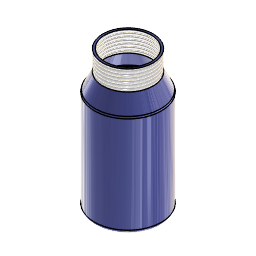
bottle_bottom (Autodesk Fusion 360 archive; units mm, degrees)
design "bottle_bottom" references "hhhhhhh"
part number: 2025-09-29-05-59-28-951
Autodesk Fusion 360 part; units mm, degrees
sketch "Sketch1" plane through (0, 0, 0) normal (0, 0, 1) x (1, 0, 0)
  circle A0 centre (0, 0) radius 16.5
  dimension "d1" = 33
  constraint coincident A0.centre origin
  measures "d1" diameter of A0
extrude "Extrude1" add sketch "Sketch1" along normal blind 50
ref_plane "WorkPlane1" through (0, 0, 55) normal (0, 0, 1) x (1, 0, 0)
sketch "Sketch2" plane through (0, 0, 55) normal (0, 0, 1) x (1, 0, 0)
  circle A0 centre (0, 0) radius 12.5
  dimension "d5" = 25
  constraint coincident A0.centre origin
  measures "d5" diameter of A0
ref_plane "WorkPlane2" through (0, 0, 58) normal (0, 0, 1) x (1, 0, 0)
sketch "Sketch3" plane through (0, 0, 58) normal (0, 0, 1) x (1, 0, 0)
  circle A0 centre (0, 0) radius 12.5
  dimension "d9" = 25
  constraint coincident A0.centre origin
  measures "d9" diameter of A0
loft "Loft2" add profiles "Sketch3" section 1 face at (-4.5443, 3.0983, 50) section 2
extrude "Extrude3" add 1 faces at (-3.3879, -0.621, 58) along direction (0, 0, 1) blind 10
thread "Thread1" "ISO Metric profile 25.0 M25x1.5 M25x1.5 6g" major diameter 24.85 minor diameter 23.132 pitch 1.5 angle 60 resizes the face on face at (12.4845, -0.6231, 64.6667)
fillet "Fillet1" radius 2 2 edges at (-15.3834, -5.9667, 50) (-15.3834, -5.9667, 0)
shell "Shell1" thickness 1 removed faces 1 at (-1.595, 5.7536, 68)

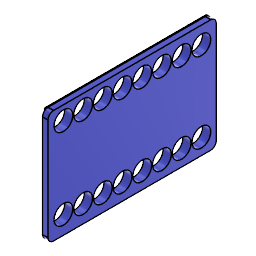
design "hhhhhhh"
part number: 2025-09-26-13-29-13-147
Autodesk Fusion 360 part; units mm, degrees
sketch "Sketch1" plane through (0, 0, 0) normal (1, 0, 0) x (0, 1, 0)
  line L0 (-10, 0) -> (-295, 0)
  line L1 (-305, 10) -> (-305, 195)
  line L2 (-295, 205) -> (-10, 205)
  line L3 (0, 195) -> (0, 10)
  circle A0 centre (-27, 174) radius 17
  circle A1 centre (-62.7143, 175) radius 17
  circle A2 centre (-98.4283, 176) radius 17
  circle A3 centre (-134.1423, 177) radius 17
  circle A4 centre (-169.8563, 178) radius 17
  circle A5 centre (-205.5703, 179) radius 17
  circle A6 centre (-241.2843, 179.5) radius 17
  circle A7 centre (-276.9983, 180) radius 17
  circle A8 centre (-27, 29) radius 17
  circle A9 centre (-62.7127, 29.3029) radius 17
  circle A10 centre (-98.4267, 29.6) radius 17
  circle A11 centre (-134.1407, 29.9) radius 17
  circle A12 centre (-169.8547, 30.1) radius 17
  circle A13 centre (-205.5687, 31) radius 17
  circle A14 centre (-241.2827, 32) radius 17
  arc A15 (-305, 10) -> (-295, 0) centre (-295, 10) ccw
  arc A16 (-295, 205) -> (-305, 195) centre (-295, 195) ccw
  arc A17 (0, 195) -> (-10, 205) centre (-10, 195) ccw
  arc A18 (-10, 0) -> (0, 10) centre (-10, 10) ccw
  circle A19 centre (-276.9967, 33) radius 17
  dimension "d1" = 305
  dimension "d2" = 205
  dimension "d3" = 34
  dimension "d4" = 27
  dimension "d5" = 31
  dimension "d6" = 34
  dimension "d7" = 34
  dimension "d8" = 34
  dimension "d9" = 34
  dimension "d10" = 34
  dimension "d11" = 35.7143
  dimension "d12" = 35.714
  dimension "d13" = 35.714
  dimension "d14" = 35.714
  dimension "d15" = 35.714
  dimension "d16" = 34
  dimension "d17" = 34
  dimension "d18" = 35.714
  dimension "d19" = 35.714
  dimension "d20" = 28.0017
  dimension "d21" = 34
  dimension "d22" = 34
  dimension "d23" = 34
  dimension "d24" = 34
  dimension "d25" = 34
  dimension "d26" = 34
  dimension "d27" = 34
  dimension "d28" = 27
  dimension "d29" = 35.714
  dimension "d30" = 35.714
  dimension "d31" = 10
  dimension "d32" = 10
  dimension "d33" = 10
  dimension "d34" = 10
  dimension "d35" = 35.714
  dimension "d36" = 35.714
  dimension "d37" = 35.714
  dimension "d38" = 35.714
  dimension "d39" = 34
  dimension "d40" = 35.714
  dimension "d41" = 28.0033
  dimension "d42" = 29
  dimension "d44" = 29.6
  dimension "d45" = 29.3029
  dimension "d46" = 29.9
  dimension "d47" = 30.1
  dimension "d48" = 31
  dimension "d49" = 32
  dimension "d50" = 33
  dimension "d51" = 25
  dimension "d52" = 25.5
  dimension "d53" = 26
  dimension "d54" = 27
  dimension "d55" = 28
  dimension "d56" = 29
  dimension "d57" = 30
  dimension "d58" = 31
  constraint horizontal L0
  constraint vertical L1
  constraint horizontal L2
  constraint vertical L3
  constraint tangent L0 A15
  constraint tangent L1 A15
  constraint tangent L1 A16
  constraint tangent L2 A16
  constraint tangent L3 A17
  constraint tangent L2 A17
  constraint tangent L0 A18
  constraint tangent L3 A18
  measures "d1" distance of L1 L3
  measures "d2" distance of L0 L2
  measures "d3" diameter of A0
  measures "d4" distance of L3 A0.centre
  measures "d5" distance of L2 A0.centre
  measures "d6" diameter of A1
  measures "d7" diameter of A2
  measures "d8" diameter of A3
  measures "d9" diameter of A4
  measures "d10" diameter of A5
  measures "d11" horizontal distance of A0.centre A1.centre
  measures "d12" horizontal distance of A1.centre A2.centre
  measures "d13" horizontal distance of A2.centre A3.centre
  measures "d14" horizontal distance of A3.centre A4.centre
  measures "d15" horizontal distance of A4.centre A5.centre
  measures "d16" diameter of A7
  measures "d17" diameter of A6
  measures "d18" horizontal distance of A5.centre A6.centre
  measures "d19" horizontal distance of A6.centre A7.centre
  measures "d20" distance of L1 A7.centre
  measures "d21" diameter of A8
  measures "d22" diameter of A9
  measures "d23" diameter of A10
  measures "d24" diameter of A11
  measures "d25" diameter of A12
  measures "d26" diameter of A13
  measures "d27" diameter of A14
  measures "d28" distance of L3 A8.centre
  measures "d29" distance of A8.centre A9.centre
  measures "d30" horizontal distance of A9.centre A10.centre
  measures "d31" radius of A15
  measures "d32" radius of A16
  measures "d33" radius of A17
  measures "d34" radius of A18
  measures "d35" horizontal distance of A10.centre A11.centre
  measures "d36" horizontal distance of A11.centre A12.centre
  measures "d37" horizontal distance of A12.centre A13.centre
  measures "d38" horizontal distance of A13.centre A14.centre
  measures "d39" diameter of A19
  measures "d40" horizontal distance of A14.centre A19.centre
  measures "d41" distance of L1 A19.centre
  measures "d42" distance of L0 A8.centre
  measures "d44" distance of L0 A10.centre
  measures "d45" distance of L0 A9.centre
  measures "d46" distance of L0 A11.centre
  measures "d47" distance of L0 A12.centre
  measures "d48" distance of L0 A13.centre
  measures "d49" distance of L0 A14.centre
  measures "d50" distance of L0 A19.centre
  measures "d51" distance of L2 A7.centre
  measures "d52" distance of L2 A6.centre
  measures "d53" distance of L2 A5.centre
  measures "d54" distance of L2 A4.centre
  measures "d55" distance of L2 A3.centre
  measures "d56" distance of L2 A2.centre
  measures "d57" distance of L2 A1.centre
  measures "d58" distance of L2 A0.centre
extrude "Extrude1" add sketch "Sketch1" along normal blind 10
sketch "Sketch2" plane through (0, 0, 0) normal (0, 0, 1) x (1, 0, 0)
sketch "Sketch3" plane through (0, 0, 0) normal (-1, 0, 0) x (0, -1, 0)
  circle A0 centre (169.8563, 178) radius 17
  circle A1 centre (205.5687, 31) radius 17
  circle A2 centre (98.4267, 29.6) radius 17
  circle A3 centre (134.1407, 29.9) radius 17
  circle A4 centre (62.7143, 175) radius 17
  circle A5 centre (27, 29) radius 17
  circle A6 centre (98.4283, 176) radius 17
  circle A7 centre (62.7127, 29.3029) radius 17
  circle A8 centre (134.1423, 177) radius 17
  circle A9 centre (169.8547, 30.1) radius 17
  circle A10 centre (241.2827, 32) radius 17
  circle A11 centre (241.2843, 179.5) radius 17
  circle A12 centre (276.9967, 33) radius 17
  circle A13 centre (276.9983, 180) radius 17
  circle A14 centre (27, 174) radius 17
  circle A15 centre (205.5703, 179) radius 17
  arc A16 (295, 0) -> (305, 10) centre (295, 10) ccw
  line L0 (305, 10) -> (305, 195)
  arc A17 (305, 195) -> (295, 205) centre (295, 195) ccw
  line L1 (295, 205) -> (10, 205)
  arc A18 (10, 205) -> (0, 195) centre (10, 195) ccw
  line L2 (0, 195) -> (0, 10)
  arc A19 (0, 10) -> (10, 0) centre (10, 10) ccw
  line L3 (10, 0) -> (295, 0)
  line L4 (2.9289, 202.0711) -> (296.3472, 202.0711)
  line L5 (296.3472, 202.0711) -> (296.3472, 155.653)
  line L6 (296.3472, 155.653) -> (2.9289, 155.653)
  line L7 (2.9289, 155.653) -> (2.9289, 202.0711)
  line L8 (6.0644, 54.9839) -> (296.0644, 54.9839)
  line L9 (296.0644, 54.9839) -> (296.0644, 10)
  line L10 (296.0644, 10) -> (6.0644, 10)
  line L11 (6.0644, 10) -> (6.0644, 54.9839)
  dimension "d61" = 290
  constraint horizontal L4
  constraint vertical L5
  constraint horizontal L6
  constraint vertical L7
  constraint midpoint A18 L4.start
  constraint horizontal L8
  constraint vertical L9
  constraint horizontal L10
  constraint vertical L11
  measures "d61" distance of L8.start L8.end
extrude "Extrude2" add sketch "Sketch3" along normal blind 5 contours L4 L5 L6 L7 | L8 L9 L10 L11
sketch "Sketch4" plane through (10, 0, 0) normal (1, 0, 0) x (0, 1, 0)
  circle A0 centre (-169.8563, 178) radius 17
  circle A1 centre (-205.5687, 31) radius 17
  circle A2 centre (-98.4267, 29.6) radius 17
  circle A3 centre (-134.1407, 29.9) radius 17
  circle A4 centre (-62.7143, 175) radius 17
  circle A5 centre (-27, 29) radius 17
  circle A6 centre (-98.4283, 176) radius 17
  circle A7 centre (-62.7127, 29.3029) radius 17
  circle A8 centre (-134.1423, 177) radius 17
  circle A9 centre (-169.8547, 30.1) radius 17
  circle A10 centre (-241.2827, 32) radius 17
  circle A11 centre (-241.2843, 179.5) radius 17
  circle A12 centre (-276.9967, 33) radius 17
  circle A13 centre (-276.9983, 180) radius 17
  circle A14 centre (-27, 174) radius 17
  circle A15 centre (-205.5703, 179) radius 17
  arc A16 (-305, 10) -> (-295, 0) centre (-295, 10) ccw
  line L0 (-295, 0) -> (-10, 0)
  arc A17 (-10, 0) -> (0, 10) centre (-10, 10) ccw
  line L1 (0, 10) -> (0, 195)
  arc A18 (0, 195) -> (-10, 205) centre (-10, 195) ccw
  line L2 (-10, 205) -> (-295, 205)
  arc A19 (-295, 205) -> (-305, 195) centre (-295, 195) ccw
  line L3 (-305, 195) -> (-305, 10)
  line L4 (-295, 205) -> (-24.7534, 205)
  line L5 (-24.7534, 205) -> (-24.7534, 197.6073)
  line L6 (-24.7534, 197.6073) -> (-295, 197.6073)
  line L7 (-295, 197.6073) -> (-295, 205)
  line L8 (-290, 10) -> (-20.1383, 10)
  line L9 (-20.1383, 10) -> (-20.1383, 2.9289)
  line L10 (-20.1383, 2.9289) -> (-290, 2.9289)
  line L11 (-290, 2.9289) -> (-290, 10)
  line L12 (-305, 177.0494) -> (-294.5229, 177.0494)
  line L13 (-294.5229, 177.0494) -> (-294.5229, 46.9894)
  line L14 (-294.5229, 46.9894) -> (-305, 46.9894)
  line L15 (-305, 46.9894) -> (-305, 177.0494)
  line L16 (-10, 160) -> (0, 160)
  line L17 (0, 160) -> (0, 40)
  line L18 (0, 40) -> (-10, 40)
  line L19 (-10, 40) -> (-10, 160)
  constraint horizontal L4
  constraint vertical L5
  constraint horizontal L6
  constraint vertical L7
  constraint coincident L2.end A19.start
  constraint horizontal L8
  constraint vertical L9
  constraint horizontal L10
  constraint vertical L11
  constraint horizontal L12
  constraint vertical L13
  constraint horizontal L14
  constraint vertical L15
  constraint coincident L3 L12.start
  constraint horizontal L16
  constraint vertical L17
  constraint horizontal L18
  constraint vertical L19
sketch "Sketch5" plane through (0, 0, 0) normal (-1, 0, 0) x (0, -1, 0)
  arc A0 (295, 0) -> (305, 10) centre (295, 10) ccw
  line L0 (305, 10) -> (305, 195)
  arc A1 (305, 195) -> (295, 205) centre (295, 195) ccw
  line L1 (295, 205) -> (10, 205)
  arc A2 (10, 205) -> (2.9289, 202.0711) centre (10, 195) ccw
  line L2 (2.9289, 202.0711) -> (296.3472, 202.0711)
  line L3 (296.3472, 202.0711) -> (296.3472, 155.653)
  line L4 (296.3472, 155.653) -> (2.9289, 155.653)
  line L5 (2.9289, 155.653) -> (2.9289, 202.0711)
  line L6 (0, 195) -> (0, 10)
  arc A3 (0, 10) -> (10, 0) centre (10, 10) ccw
  line L7 (10, 0) -> (295, 0)
  line L8 (6.0644, 10) -> (6.0644, 54.9839)
  line L9 (6.0644, 54.9839) -> (296.0644, 54.9839)
  line L10 (296.0644, 54.9839) -> (296.0644, 10)
  line L11 (296.0644, 10) -> (6.0644, 10)
  line L12 (0, 110) -> (30, 110)
  line L13 (30, 110) -> (30, 0)
  line L14 (30, 0) -> (0, 0)
  line L15 (0, 0) -> (0, 110)
  line L16 (110, 0) -> (-0.4275, 0)
  line L17 (-0.4275, 0) -> (-0.4275, 54.9839)
  line L18 (-0.4275, 54.9839) -> (110, 54.9839)
  line L19 (110, 54.9839) -> (110, 0)
  arc A4 (2.9289, 202.0711) -> (0, 195) centre (10, 195) ccw
  constraint horizontal L12
  constraint vertical L13
  constraint horizontal L14
  constraint vertical L15
  constraint coincident L6 L12.start
  constraint horizontal L16
  constraint vertical L17
  constraint horizontal L18
  constraint vertical L19
  constraint coincident L7 L16.start
